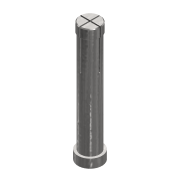
# Autodesk Inventor part: Pin_Dedao
Saved by Autodesk Inventor 2020 (Build 240168000, 168)
## iProperties
Created: 2021-04-01
Part Number: Pin_Dedao
Material: Generic
Document SubType Name: Modeling
Designer: deox
Density: 1 g/cm^3
Appearance: Galvanized
Author: deox
Autodesk Inventor part; units mm, degrees
ref_plane "YZ Plane" through (0, 0, 0) normal (1, 0, 0) x (0, 1, 0)
ref_plane "XZ Plane" through (0, 0, 0) normal (0, 1, 0) x (-1, 0, 0)
ref_plane "XY Plane" through (0, 0, 0) normal (0, 0, 1) x (1, 0, 0)
sketch "Sketch1" plane through (0, 0, 0) normal (0, 1, 0) x (-1, 0, 0)
  circle A0 centre (0, 0) radius 0.825
  dimension "d0" = 1.65
  constraints: 1 centre point, 1 coincident
  measures "d0" diameter of A0
extrude "Extrusion1" add sketch "Sketch1" along normal blind 0.605
sketch "Sketch2" plane through (0, 0.605, 0) normal (0, 1, 0) x (1, 0, 0)
  circle A0 centre (0, 0) radius 0.825 projected
  circle A1 centre (0, 0) radius 0.66
  dimension "d3" = 1.32
  constraints: 1 centre point, 1 coincident
  measures "d3" diameter of A1
extrude "Extrusion2" add sketch "Sketch2" along normal blind 6.96 contours A1
sketch "Sketch3" plane through (0, 7.565, 0) normal (0, 1, 0) x (1, 0, 0)
  circle A0 centre (0, 0) radius 0.715
  dimension "d6" = 1.43
  constraints: 1 centre point, 1 coincident
  measures "d6" diameter of A0
extrude "Extrusion3" add sketch "Sketch3" along normal blind 0.6875
chamfer "Chamfer1" distance 0.055 angle 45 2 edges at (-0.715, 8.2525, 0) (-0.715, 7.565, 0)
sketch "Sketch4" plane through (0, 0, 0) normal (0, 0, 1) x (1, 0, 0)
  line L0 (-0.66, 8.2525) -> (0.66, 8.2525) projected
  line L1 (0, 8.2525) -> (0.0412, 8.2525)
  line L2 (0.0412, 8.2525) -> (0.0412, 5.5025)
  line L3 (0.0412, 5.5025) -> (0, 5.5025)
  circle A0 centre (0, 5.5025) radius 0.0412
  line L4 (0, 5.5025) -> (0, 5.524)
  line L5 (-0.0412, 8.2525) -> (-0.0412, 5.5025)
  line L6 (-0.0412, 8.2525) -> (0, 8.2525)
  point P0 (0, 0)
  dimension "d12" = 0.0413
  dimension "d13" = 2.75
  constraints: 12 end point, 2 symmetric about line, 2 vertical, 1 coincident, 1 collinear, 1 horizontal, 1 midpoint, 1 point on line, 3 other
  measures "d12" distance of L1.start L1.end
  measures "d13" distance of L1.end L2.end
extrude "Extrusion4" cut sketch "Sketch4" against normal mid plane 2.1875
pattern_circular "Circular Pattern1" count 4 over 360 about axis through (0, 0.605, 0) along (0, 1, 0) of "Extrusion4"
body "Solid1"
